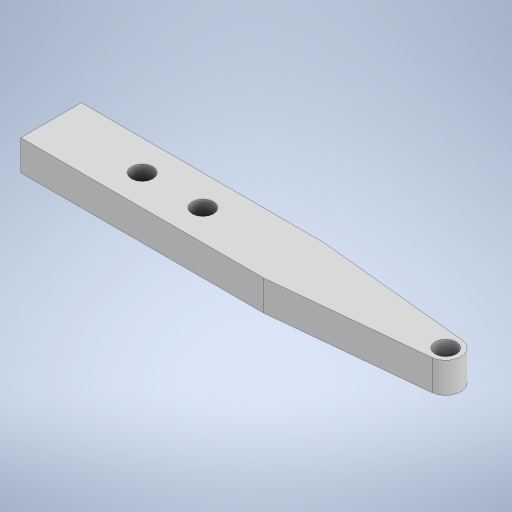
# Autodesk Inventor part: 4-bar intake block
Saved by Autodesk Inventor 2023 (Build 270158030, 158C)
## iProperties
Created: 2022-07-18
Part Number: 4-bar intake block
Material: Generic
Document SubType Name: Modeling
Designer: kt1040502
Density: 1 g/cm^3
Appearance: Default
Author: kt1040502
Autodesk Inventor part; units mm, degrees
ref_plane "YZ Plane" through (0, 0, 0) normal (1, 0, 0) x (0, 1, 0)
ref_plane "XZ Plane" through (0, 0, 0) normal (0, 1, 0) x (-1, 0, 0)
ref_plane "XY Plane" through (0, 0, 0) normal (0, 0, 1) x (1, 0, 0)
sketch "Sketch1" plane through (0, 0, 0) normal (0, 1, 0) x (-1, 0, 0)
  line L0 (0, 0) -> (-203.2, 0)
  line L1 (0, 25.4) -> (-76.2, 25.4) construction
  line L2 (-203.2, 25.4) -> (-127, 25.4) construction
  line L3 (-127, 25.4) -> (-330.2, 25.4)
  circle A0 centre (-330.2, 25.4) radius 12.7
  circle A1 centre (-76.2, 25.4) radius 8.89
  circle A2 centre (-127, 25.4) radius 8.89
  line L4 (0, 0) -> (-203.2, 0)
  line L5 (-203.2, 50.8) -> (0, 50.8)
  line L6 (0, 50.8) -> (0, 0)
  line L7 (-203.2, 50.8) -> (-331.4575, 38.0376)
  line L8 (-203.2, 0) -> (-331.4575, 12.7624)
  circle A3 centre (-330.2, 25.4) radius 8.89
  dimension "d2" = 76.2
  dimension "d3" = 76.2
  dimension "d8" = 203.2
  dimension "d9" = 25.4
  dimension "d10" = 17.78
  dimension "d11" = 17.78
  dimension "d12" = 50.8
  dimension "d13" = 17.78
  constraints: 18 end point, 5 coincident, 5 horizontal, 4 centre point, 2 point on circle, 2 tangent, 1 parallel
  measures "d2" distance of L1.start L1.end
  measures "d3" distance of L2.start L2.end
  measures "d8" distance of L3.start L3.end
  measures "d9" diameter of A0
  measures "d10" diameter of A1
  measures "d11" diameter of A2
  measures "d12" distance of L4.end L5.start
  measures "d13" diameter of A3
extrude "Extrusion1" add sketch "Sketch1" along normal blind 25.4
body "Solid1"
